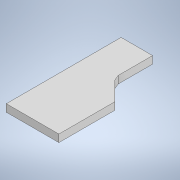
# Autodesk Inventor part: VerstaerkungHintenLinks
Saved by Autodesk Inventor 2020.3 (Build 243373010, 373A)
## iProperties
Created: 2021-02-13
Part Number: VerstaerkungHintenLinks
Material: Generisch
Document SubType Name: Modeling
Designer: Stefan
Density: 1 g/cm^3
Appearance: Vorgabe
Author: Stefan
Autodesk Inventor part; units mm, degrees
ref_plane "YZ Plane" through (0, 0, 0) normal (1, 0, 0) x (0, 1, 0)
ref_plane "XZ Plane" through (0, 0, 0) normal (0, 1, 0) x (-1, 0, 0)
ref_plane "XY Plane" through (0, 0, 0) normal (0, 0, 1) x (1, 0, 0)
sketch "Skizze1" plane through (0, 0, 0) normal (0, 1, 0) x (-1, 0, 0)
  line L0 (100.9437, 169.5604) -> (-41.0563, 169.5604)
  line L1 (-41.0563, 169.5604) -> (-41.0563, -140.4396)
  line L2 (-41.0563, -140.4396) -> (100.9437, -140.4396)
  line L3 (100.9437, -140.4396) -> (100.9437, 169.5604)
  line L4 (43.9437, 169.5604) -> (43.9437, -140.4396) construction
  point P0 (0, 0)
  dimension "d0" = 142
  dimension "d1" = 310
  dimension "d3" = 85
  constraints: 10 end point, 2 parallel, 2 perpendicular, 2 point on line, 1 horizontal, 1 other
  measures "d0" distance of L1.end L2.end
  measures "d1" distance of L0.end L1.end
  measures "d3" distance between parallel lines of L1 L4
extrude "Extrusion1" add sketch "Skizze1" along normal blind 20
sketch "Skizze2" plane through (0, 20, 0) normal (0, 1, 0) x (1, 0, 0)
  line L0 (-105.9437, 300.3701) -> (-105.9437, -171.184)
  line L1 (-105.9437, -171.184) -> (-105.45, -169.5604)
  line L2 (-105.45, -169.5604) -> (711.1561, -169.5604)
  line L3 (711.1561, -169.5604) -> (855.4636, -169.5604)
  line L4 (377.6538, -128.0898) -> (230.4587, -128.0898)
  line L5 (230.4587, -128.0898) -> (94.4681, -71.7607)
  line L6 (94.4681, -71.7607) -> (-9.6146, 32.322)
  line L7 (-9.6146, 32.322) -> (-65.9437, 168.3126)
  line L8 (-65.9437, 168.3126) -> (-65.9437, 315.5078)
  line L9 (-100.9437, -169.5604) -> (41.0563, -169.5604) projected
  line L10 (-100.9437, 140.4396) -> (-100.9437, -169.5604) projected
  line L11 (-65.9437, 168.3126) -> (145.1779, 204.9795)
  line L12 (145.1779, 204.9795) -> (211.023, 17.308)
  line L13 (211.023, 17.308) -> (94.4681, -71.7607)
  line L14 (-15.9437, -169.5604) -> (-15.9437, 176.9964)
  line L15 (41.0563, 140.4396) -> (-100.9437, 140.4396) projected
  point P0 (0, 0)
  point P1 (-15.9437, 47.6019)
  dimension "d3" = 85
  dimension "d44" = 147.1952
  dimension "d45" = 147.1952
  dimension "d46" = 147.1952
  dimension "d48" = 147.1952
  dimension "d49" = 147.1952
  dimension "d50" = 816.6061
  dimension "d52" = 471.5541
  dimension "d53" = 40
  dimension "d54" = 1.697
  dimension "d55" = 90
  dimension "d56" = 157.5
  dimension "d57" = 157.5
  dimension "d58" = 157.5
  dimension "d60" = 41.4706
  dimension "d61" = 0
  dimension "d62" = 5
  dimension "d63" = 85
  constraints: 26 end point, 2 perpendicular, 2 point on line, 1 horizontal, 1 parallel, 1 vertical
  measures "d44" distance of L7.end L8.end
  measures "d45" distance of L6.end L7.end
  measures "d46" distance of L5.end L6.end
  measures "d48" distance of L4.end L5.end
  measures "d49" distance of L4.start L4.end
  measures "d50" distance of L1.end L2.end
  measures "d52" distance of L0.start L0.end
  measures "d53" distance between parallel lines of L8 L0
  measures "d54" distance of L0.end L1.end
  measures "d55" angle of L0 L2
  measures "d56" angle of L8 L7
  measures "d57" angle of L6 L7
  measures "d58" angle of L6 L5
  measures "d60" distance from line of L2 L4.start
  measures "d61" distance between parallel lines of L9 L2
  measures "d62" distance from line of L0.start L10
  measures "d63" distance between parallel lines of L10 L14
extrude "Extrusion2" cut sketch "Skizze2" against normal through all contours L14 L11 L12 L13 L6 L7
